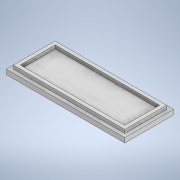
# Autodesk Inventor part: Wireless charger Cover
Saved by Autodesk Inventor 2020 (Build 240168000, 168)
## iProperties
Created: 2020-03-22
Part Number: Wireless charger Cover
Material: Generic
Document SubType Name: Modeling
Designer: Admin
Density: 1 g/cm^3
Appearance: Default
Author: Admin
Autodesk Inventor part; units mm, degrees
ref_plane "YZ Plane" through (0, 0, 0) normal (1, 0, 0) x (0, 1, 0)
ref_plane "XZ Plane" through (0, 0, 0) normal (0, 1, 0) x (-1, 0, 0)
ref_plane "XY Plane" through (0, 0, 0) normal (0, 0, 1) x (1, 0, 0)
sketch "Sketch1" plane through (0, 0, 0) normal (0, 1, 0) x (-1, 0, 0)
  line L0 (0, 0) -> (170, 0)
  line L1 (170, 0) -> (170, -70)
  line L2 (170, -70) -> (0, -70)
  line L3 (0, -70) -> (0, 0)
  dimension "d0" = 170
  dimension "d1" = 70
  constraints: 8 end point, 2 parallel, 1 horizontal, 1 perpendicular
  measures "d0" distance of L1.end L2.end
  measures "d1" distance of L0.end L1.end
extrude "Extrusion1" add sketch "Sketch1" along normal blind 7
sketch "Sketch2" plane through (0, 7, 0) normal (0, 1, 0) x (1, 0, 0)
  line L0 (-165, 5) -> (-5, 5)
  line L1 (-5, 5) -> (-5, 65)
  line L2 (-5, 65) -> (-165, 65)
  line L3 (-165, 65) -> (-165, 5)
  line L4 (-170, 70) -> (-170, 0) projected
  line L5 (0, 70) -> (-170, 70) projected
  line L6 (0, 0) -> (0, 70) projected
  line L7 (-170, 0) -> (0, 0) projected
  line L8 (-160, 10) -> (-10, 10)
  line L9 (-10, 10) -> (-10, 60)
  line L10 (-10, 60) -> (-160, 60)
  line L11 (-160, 60) -> (-160, 10)
  dimension "d4" = 5
  dimension "d5" = 5
  dimension "d6" = 5
  dimension "d7" = 5
  dimension "d8" = 5
  dimension "d9" = 5
  dimension "d10" = 5
  dimension "d11" = 5
  constraints: 16 end point, 4 parallel, 2 horizontal, 2 perpendicular
  measures "d4" distance between parallel lines of L4 L3
  measures "d5" distance between parallel lines of L5 L2
  measures "d6" distance between parallel lines of L6 L1
  measures "d7" distance between parallel lines of L7 L0
  measures "d8" distance between parallel lines of L3 L11
  measures "d9" distance between parallel lines of L2 L10
  measures "d10" distance between parallel lines of L1 L9
  measures "d11" distance between parallel lines of L0 L8
extrude "Extrusion2" add sketch "Sketch2" along normal blind 5 contours L3 L2 L1 L0
body "Solid1"
